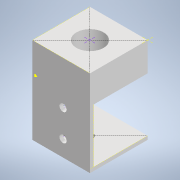
# Autodesk Inventor part: Bearing Housing
Saved by Autodesk Inventor 2020 (Build 240168000, 168)
## iProperties
Created: 2021-12-14
Part Number: Bearing Housing
Material: Generic
Document SubType Name: Modeling
Designer: danie
Density: 1 g/cm^3
Appearance: Default
Author: danie
Autodesk Inventor part; units mm, degrees
ref_plane "YZ Plane" through (0, 0, 0) normal (1, 0, 0) x (0, 1, 0)
ref_plane "XZ Plane" through (0, 0, 0) normal (0, 1, 0) x (-1, 0, 0)
ref_plane "XY Plane" through (0, 0, 0) normal (0, 0, 1) x (1, 0, 0)
sketch "Sketch1" plane through (0, 0, 0) normal (0, 1, 0) x (-1, 0, 0)
  line L0 (0, 0) -> (50.8, 0)
  line L1 (50.8, 0) -> (50.8, -50.8)
  line L2 (50.8, -50.8) -> (0, -50.8)
  line L3 (0, -50.8) -> (0, 0)
  line L4 (47.625, -3.175) -> (3.175, -3.175)
  line L5 (3.175, -3.175) -> (3.175, -47.625)
  line L6 (3.175, -47.625) -> (47.625, -47.625)
  line L7 (47.625, -47.625) -> (47.625, -3.175)
  line L8 (47.625, -47.625) -> (47.625, -50.8)
  line L9 (3.175, -3.175) -> (0, -3.175)
  dimension "d0" = 50.8
  dimension "d1" = 50.8
  dimension "d2" = 3.175
  constraints: 20 end point, 4 parallel, 4 perpendicular, 2 point on line, 1 horizontal, 3 other
  measures "d0" distance of L1.end L2.end
  measures "d1" distance of L0.end L1.end
  measures "d2" distance between parallel lines of L0 L4
extrude "Extrusion1" add sketch "Sketch1" against normal blind 25.4 contours L0 L1 L2 L8 L7 L4 L9 L3
sketch "Sketch2" plane through (0, 0, 0) normal (0, 1, 0) x (1, 0, 0)
  line L0 (-50.8, 0) -> (-50.8, 50.8) projected
  line L1 (-50.8, 0) -> (0, 0)
  line L2 (0, 0) -> (0, 50.8)
  line L3 (0, 50.8) -> (-50.8, 50.8)
  line L4 (-50.8, 50.8) -> (-50.8, 0)
  dimension "d5" = 50.8
  constraints: 8 end point, 2 parallel, 1 horizontal, 1 perpendicular
  measures "d5" distance of L2.end L1.end
extrude "Extrusion2" add sketch "Sketch2" along normal blind 25.4
sketch "Sketch3" plane through (0, 25.4, 0) normal (0, 1, 0) x (1, 0, 0)
  line L0 (-50.8, 0) -> (-50.8, 50.8) construction
  line L1 (-50.8, 0) -> (0, 50.8) construction
  line L2 (0, 0) -> (-50.8, 0) construction
  line L3 (0, 0) -> (-50.8, 50.8) construction
  point P0 (-25.61, 25.3161)
  constraints: 4 end point
sketch "Sketch4" plane through (0, 25.4, 0) normal (0, 1, 0) x (1, 0, 0)
  point P0 (0, 0)
  point P1 (-25.3999, 25.4)
hole "Hole1" at (-25.3999, 25.4, -25.4) direction (0, -1, 0) diameter 25.4 end through all
sketch "Sketch5" plane through (0, -25.4, -3.175) normal (0, 0, -1) x (-1, 0, 0)
  line L0 (0, 25.4) -> (0, 0) construction
  line L1 (47.625, 0) -> (0, 0) construction
  line L2 (0, 25.4) -> (47.625, 0) construction
  line L3 (0, 25.4) -> (47.625, 25.4) construction
  line L4 (0, 0) -> (47.625, 25.4) construction
  constraints: 4 end point
sketch "Sketch6" plane through (0, -25.4, -3.175) normal (0, 0, -1) x (-1, 0, 0)
  point P0 (0, 25.4)
  point P1 (23.8125, 12.7)
hole "Hole2" at (-23.8125, -12.7, -3.175) direction (0, 0, 1) diameter 6.35 end through all
sketch "Sketch7" plane through (-47.625, -25.4, -3.175) normal (1, 0, 0) x (0, 0, -1)
  line L0 (47.625, 0) -> (0, 0) construction
  line L1 (0, 25.4) -> (0, 0) construction
  line L2 (47.625, 0) -> (0, 25.4) construction
  line L3 (47.625, 25.4) -> (47.625, 0) construction
  line L4 (0, 0) -> (47.625, 25.4) construction
  point P0 (-3.175, 25.4)
  constraints: 4 end point
sketch "Sketch8" plane through (-47.625, -25.4, -3.175) normal (1, 0, 0) x (0, 0, -1)
  point P0 (-3.175, 25.4)
  point P1 (23.8116, 12.6997)
hole "Hole3" at (-47.625, -12.7003, -26.9866) direction (-1, 0, 0) diameter 6.35 end through all
sketch "Sketch9" plane through (0, -25.4, 0) normal (0, -1, 0) x (1, 0, 0)
  line L0 (-50.8, -50.8) -> (-50.8, 0) projected
  line L1 (0, 0) -> (-50.8, 0)
  line L2 (-50.8, 0) -> (-50.8, -50.8)
  line L3 (-50.8, -50.8) -> (0, -50.8)
  line L4 (0, -50.8) -> (0, 0)
  line L5 (-47.625, -3.175) -> (-3.175, -3.175)
  line L6 (-3.175, -3.175) -> (-3.175, -47.625)
  line L7 (-3.175, -47.625) -> (-47.625, -47.625)
  line L8 (-47.625, -47.625) -> (-47.625, -3.175)
  line L9 (0, -3.175) -> (-47.625, -3.175) projected
  line L10 (-3.175, -3.175) -> (0, -3.175)
  line L11 (-47.625, -47.625) -> (-47.625, -50.8)
  point P0 (-3.175, -3.175)
  constraints: 20 end point, 4 parallel, 2 horizontal, 2 perpendicular, 1 point on line, 1 vertical, 3 other
extrude "Extrusion3" add sketch "Sketch9" along normal blind 25.4 contours L0 L1 L4 L9 L5 L8 L11 L3
sketch "Sketch10" plane through (0, -50.8, 0) normal (0, -1, 0) x (1, 0, 0)
  line L0 (0, 0) -> (-50.8, 0)
  line L1 (-50.8, 0) -> (-50.8, -50.8)
  line L2 (-50.8, -50.8) -> (0, -50.8)
  line L3 (0, -50.8) -> (0, 0)
  constraints: 8 end point, 2 parallel, 1 horizontal, 1 perpendicular
extrude "Extrusion4" add sketch "Sketch10" against normal blind 3.175
sketch "Sketch11" plane through (0, 0, -3.175) normal (0, 0, -1) x (-1, 0, 0)
  line L0 (47.625, 0) -> (47.625, -47.625) construction
  line L1 (47.625, -47.625) -> (0, -25.4001) construction
  line L2 (0, 0) -> (0, -47.625) construction
  line L3 (0, -47.625) -> (47.625, -47.625) construction
  line L4 (47.625, -25.4001) -> (0, -47.625) construction
  constraints: 4 end point, 1 point on line
sketch "Sketch12" plane through (0, 0, -3.175) normal (0, 0, -1) x (-1, 0, 0)
  point P0 (0, 0)
  point P1 (23.8112, -36.5118)
hole "Hole4" at (-23.8112, -36.5118, -3.175) direction (0, 0, 1) diameter 6.35 end through all
sketch "Sketch13" plane through (-47.625, 0, -3.175) normal (1, 0, 0) x (0, 0, -1)
  line L0 (0, 0) -> (0, -47.625) construction
  line L1 (0, -47.625) -> (47.625, -47.625) construction
  line L2 (0, -25.4031) -> (47.625, -47.625) construction
  line L3 (0, -47.625) -> (47.625, -25.4031) construction
  line L4 (47.625, 0) -> (47.625, -47.625) construction
  point P0 (-3.175, 0)
  constraints: 4 end point, 2 point on line
sketch "Sketch14" plane through (-47.625, 0, -3.175) normal (1, 0, 0) x (0, 0, -1)
  point P0 (-3.175, 0)
  point P1 (23.8113, -36.5122)
hole "Hole5" at (-47.625, -36.5122, -26.9863) direction (-1, 0, 0) diameter 6.35 end through all
sketch "Sketch15" plane through (0, -47.625, 0) normal (0, 1, 0) x (1, 0, 0)
  line L0 (-50.8, 0) -> (-50.8, 50.8) construction
  line L1 (0, 0) -> (-50.8, 50.8) construction
  line L2 (0, 0) -> (0, 50.8) construction
  line L3 (-50.8, 0) -> (0, 50.8) construction
  constraints: 4 end point
sketch "Sketch16" plane through (0, -47.625, 0) normal (0, 1, 0) x (1, 0, 0)
  point P0 (0, 0)
  point P1 (-25.4077, 25.4046)
hole "Hole6" at (-25.4077, -47.625, -25.4046) direction (0, -1, 0) diameter 6.35 end through all
body "Solid1"
